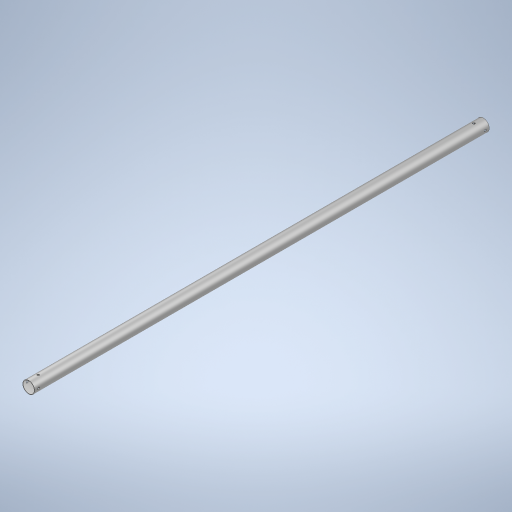
# Autodesk Inventor part: tubo Perforado
Saved by Autodesk Inventor 2024 (Build 280153000, 153)
## iProperties
RuleStatus: InUse
Created: 2026-01-02
Part Number: tubo Perforado
Material: Generic
Document SubType Name: Modeling
Designer: eduso
Density: 1 g/cm^3
Appearance: Default
Description: TB_BASE
Mass: 1598.07 g
Surface Area: 692.156 cm^2
Volume: 203.575 cm^3
AfterAnyUserParamChange0: 01_Validar_Tubo
AfterAnyUserParamChange1: 01_Validar_Tubo
AfterAnyUserParamChange2: 01_Validar_Tubo
Largo: 2890,000 mm
DiametroExterior: 76,100 mm
Espesor: 3,200 mm
DiametroInterior: 69,700 mm
Author: eduso
Autodesk Inventor part; units mm, degrees
ref_plane "XZ Plane" through (0, 0, 0) normal (0, 1, 0) x (-1, 0, 0)
ref_plane "XY Plane" through (0, 0, 0) normal (0, 0, 1) x (1, 0, 0)
sketch "Sketch1" plane through (0, 0, 0) normal (0, 0, 1) x (1, 0, 0)
  point P0 (0, 0)
sketch "Sketch2" plane through (0, 0, 0) normal (0, 0, 1) x (1, 0, 0)
  circle A0 centre (0, 0) radius 34.85
  circle A1 centre (0, 0) radius 38.05
  dimension "d0" = 76.1
  dimension "d1" = 69.7
  constraints: 2 centre point, 2 coincident
  measures "d0" diameter of A1
  measures "d1" diameter of A0
extrude "Extrusion1" add sketch "Sketch2" along normal blind 2890
sketch "Sketch3" plane through (0, 0, 0) normal (1, 0, 0) x (0, 1, 0)
  circle A0 centre (0, 25) radius 7
  line L0 (31.95, 1445) -> (-38.05, 1445)
  line L1 (-38.05, 0) -> (-38.05, 2890) projected
  circle A1 centre (0, 2865) radius 7
  line L2 (38.05, 0) -> (-38.05, 0) projected
  point P0 (0, 0)
  dimension "d7" = 25
  constraints: 2 centre point, 2 end point, 1 midpoint, 1 symmetric about line, 1 other
  measures "d7" distance from line of L2 A0.centre
extrude "Extrusion2" cut sketch "Sketch3" along normal mid plane 100
sketch "Sketch4" plane through (0, 0, 0) normal (0, 1, 0) x (-1, 0, 0)
  circle A0 centre (0, 60) radius 7
  line L0 (38.05, 0) -> (-38.05, 0) projected
  line L1 (31.95, 1445) -> (-38.05, 1445)
  line L2 (-38.05, 0) -> (-38.05, 2890) projected
  circle A1 centre (0, 2830) radius 7
  point P0 (0, 0)
  dimension "d8" = 14
  dimension "d9" = 60
  constraints: 2 centre point, 2 end point, 1 midpoint, 1 symmetric about line, 1 other
  measures "d8" diameter of A0
  measures "d9" distance from line of A0.centre L0
extrude "Extrusion3" cut sketch "Sketch4" along normal mid plane 100
ref_plane "Work Plane1" through (30.15, 0, 0) normal (1, 0, 0) x (0, 1, 0)
ref_plane "Work Plane2" through (-30.15, 0, 0) normal (1, 0, 0) x (0, 1, 0)
equation "\"espesor_testero\" = 4"
body "Solid1"
